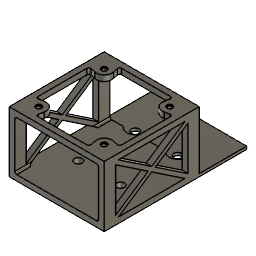
cam_support (Autodesk Fusion 360 design; units mm, degrees)
Autodesk Fusion 360 part; units mm, degrees
sketch "Esboço1" plane through (0, 0, 0) normal (0, 0, 1) x (1, 0, 0)
  line L0 (-20, 37.5) -> (20, 37.5)
  line L1 (25, 32.5) -> (25, -37.5)
  line L2 (25, -37.5) -> (-25, -37.5)
  line L3 (-25, -37.5) -> (-25, 32.5)
  line L4 (-25, 37.5) -> (25, -37.5) construction
  line L5 (25, 37.5) -> (-25, -37.5) construction
  line L6 (-25, 32.5) -> (-25, 37.5)
  line L7 (-20, 37.5) -> (-25, 37.5)
  line L8 (20, 37.5) -> (25, 37.5)
  line L9 (25, 32.5) -> (25, 37.5)
  dimension "d1" = 50
  dimension "d2" = 75
  constraint horizontal L0
  constraint perpendicular L0 L1
  constraint parallel L0 L2
  constraint parallel L1 L3
  constraint coincident L4 origin
  constraint coincident L5 origin
  constraint coincident L4.start L0
  constraint coincident L4.start L3
  constraint coincident L5.start L1
  constraint coincident L5.start L0
  measures "d1" distance of L1.end L2.end
  measures "d2" distance of L5.start L1.end
extrude "Extrusão1" add sketch "Esboço1" along normal blind 32
sketch "Esboço2" plane through (0, 0, 32) normal (0, 0, 1) x (-1, 0, 0)
  line L0 (-25, 37.5) -> (-25, -37.5)
  line L1 (-25, -37.5) -> (25, -37.5)
  line L2 (25, -37.5) -> (25, 37.5)
  line L3 (25, 37.5) -> (-25, 37.5)
  circle A0 centre (11.137, -15) radius 2.05
  circle A1 centre (-11.137, -15) radius 2.05
  circle A2 centre (11.137, 15) radius 2.05
  circle A3 centre (-11.137, 15) radius 2.05
  dimension "d6" = 4.1
  dimension "d7" = 4.1
  dimension "d8" = 4.1
  dimension "d9" = 4.1
  dimension "d10" = 22.274
  dimension "d11" = 13.863
  dimension "d12" = 13.863
  dimension "d13" = 22.274
  dimension "d14" = 30
  dimension "d15" = 22.5
  measures "d6" diameter of A0
  measures "d7" diameter of A1
  measures "d8" diameter of A2
  measures "d9" diameter of A3
  measures "d10" distance of A0.centre A1.centre
  measures "d11" distance of L2 A0.centre
  measures "d12" distance of L2 A2.centre
  measures "d13" distance of A2.centre A3.centre
  measures "d14" distance of A1.centre A3.centre
  measures "d15" distance of L1 A0.centre
extrude "Extrusão2" cut sketch "Esboço2" against normal blind 45 contours A0 | A1 | A2 | A3
ref_plane "Plano de trabalho3" through (0, 47.5, 16) normal (0, 1, 0) x (-1, 0, 0)
sketch "Esboço9" plane through (0, 47.5, 0) normal (0, 1, 0) x (-1, 0, 0)
  line L0 (-25, 0) -> (25, 0)
  line L1 (25, 0) -> (25, 32)
  line L2 (25, 32) -> (-25, 32)
  line L3 (-25, 32) -> (-25, 0)
  line L4 (16.763, 29) -> (-16.763, 29)
  line L5 (-22, 25.7693) -> (-22, 6.2307)
  line L6 (-16.763, 3) -> (16.763, 3)
  line L7 (21, 3) -> (-21, 3)
  line L8 (-22, 4) -> (-22, 28)
  line L9 (-21, 29) -> (21, 29)
  line L10 (22, 28) -> (22, 4)
  arc A0 (-21, 29) -> (-22, 28) centre (-21, 28) ccw
  arc A1 (22, 28) -> (21, 29) centre (21, 28) ccw
  arc A2 (21, 3) -> (22, 4) centre (21, 4) ccw
  arc A3 (-22, 4) -> (-21, 3) centre (-21, 4) ccw
  line L11 (-25, 0) -> (25, 0)
  line L12 (25, 0) -> (25, 32)
  line L13 (25, 32) -> (-25, 32)
  line L14 (-25, 32) -> (-25, 0)
  dimension "d156" = 1
  constraint horizontal L4
  constraint perpendicular L4 L5
  constraint parallel L4 L6
  constraint horizontal L7
  constraint perpendicular L7 L8
  constraint parallel L7 L9
  constraint parallel L8 L10
  constraint tangent L8 A0
  constraint tangent L9 A0
  constraint tangent L9 A1
  constraint tangent L10 A1
  constraint equal A0 A1
  constraint tangent L10 A2
  constraint tangent L7 A2
  constraint equal A0 A2
  constraint tangent L7 A3
  constraint tangent L8 A3
  constraint equal A0 A3
  measures "d156" radius of A0
extrude "Extrusão9" cut sketch "Esboço9" against normal blind 96 contours L4 L5 L6 L7 L8 L9 L10 A0 A1 A2 A3
sketch "Esboço12" plane through (0, 0, 32) normal (0, 0, 1) x (-1, 0, 0)
  circle A0 centre (11.137, -15) radius 2.05
  circle A1 centre (11.137, 15) radius 2.05
  circle A2 centre (-11.137, -15) radius 2.05
  circle A3 centre (-11.137, 15) radius 2.05
  line L0 (-25, 37.5) -> (-25, -37.5)
  line L1 (-25, -37.5) -> (25, -37.5)
  line L2 (25, -37.5) -> (25, 37.5)
  line L3 (25, 37.5) -> (-25, 37.5)
  line L4 (21, 34.5) -> (-21, 34.5)
  line L5 (-22, 33.5) -> (-22, -33.5)
  line L6 (-21, -34.5) -> (21, -34.5)
  line L7 (22, -33.5) -> (22, 33.5)
  line L8 (22, 34.5) -> (-22, -34.5) construction
  line L9 (-22, 34.5) -> (22, -34.5) construction
  arc A4 (-21, 34.5) -> (-22, 33.5) centre (-21, 33.5) ccw
  arc A5 (22, 33.5) -> (21, 34.5) centre (21, 33.5) ccw
  arc A6 (21, -34.5) -> (22, -33.5) centre (21, -33.5) ccw
  arc A7 (-22, -33.5) -> (-21, -34.5) centre (-21, -33.5) ccw
  dimension "d118" = 44
  dimension "d119" = 69
  dimension "d120" = 1
  constraint horizontal L4
  constraint perpendicular L4 L5
  constraint parallel L4 L6
  constraint parallel L5 L7
  constraint coincident L8 origin
  constraint coincident L9 origin
  constraint coincident L9.start L4
  constraint coincident L9.start L5
  constraint tangent L4 A4
  constraint tangent L5 A4
  constraint coincident L8.start L7
  constraint coincident L8.start L4
  constraint tangent L7 A5
  constraint tangent L4 A5
  constraint equal A4 A5
  constraint coincident L9.end L7
  constraint coincident L9.end L6
  constraint tangent L7 A6
  constraint tangent L6 A6
  constraint equal A4 A6
  constraint coincident L8.end L6
  constraint coincident L8.end L5
  constraint tangent L6 A7
  constraint tangent L5 A7
  constraint equal A4 A7
  measures "d118" distance of L8.end L9.end
  measures "d119" distance of L9.start L8.end
  measures "d120" radius of A4
extrude "Extrusão13" cut sketch "Esboço12" against normal blind 5 contours L4 L5 L6 L7 A4 A5 A6 A7
sketch "Esboço13" plane through (0, 0, 32) normal (0, 0, 1) x (-1, 0, 0)
  line L0 (21, -34.5) -> (-21, -34.5)
  arc A0 (-22, -33.5) -> (-21, -34.5) centre (-21, -33.5) ccw
  line L1 (-22, -33.5) -> (-22, 33.5)
  arc A1 (-21, 34.5) -> (-22, 33.5) centre (-21, 33.5) ccw
  line L2 (-21, 34.5) -> (21, 34.5)
  arc A2 (22, 33.5) -> (21, 34.5) centre (21, 33.5) ccw
  line L3 (22, 33.5) -> (22, -33.5)
  arc A3 (21, -34.5) -> (22, -33.5) centre (21, -33.5) ccw
  line L4 (-25, 37.5) -> (-25, -37.5)
  line L5 (-25, -37.5) -> (25, -37.5)
  line L6 (25, -37.5) -> (25, 37.5)
  line L7 (25, 37.5) -> (-25, 37.5)
  circle A4 centre (-17.2, 29.7) radius 1.05
  line L8 (-13.8524, -8.3) -> (-13.2808, -5.5)
  circle A5 centre (-17.2, 29.7) radius 4
  arc A6 (-22, -0.3726) -> (-20.8, -1.3524) centre (-21, -0.3726) ccw
  circle A7 centre (-17.2, -4.7) radius 4
  line L9 (20.8, -1.3524) -> (18, -0.7808)
  line L10 (-22, 25.3726) -> (-22, -0.3726)
  line L11 (12.8726, 34.5) -> (-12.8726, 34.5)
  arc A8 (13.8524, 33.3) -> (12.8726, 34.5) centre (12.8726, 33.5) ccw
  line L12 (20.8, 26.3524) -> (18, 25.7808)
  arc A9 (12.8726, -9.5) -> (13.8524, -8.3) centre (12.8726, -8.5) ccw
  circle A10 centre (17.2, 29.7) radius 4
  line L13 (-20.8, -1.3524) -> (-18, -0.7808)
  arc A11 (25, 32.5) -> (20, 37.5) centre (20, 32.5) ccw
  circle A12 centre (17.2, -4.7) radius 1.05
  line L14 (0, -15) -> (0, 40)
  line L15 (-13.8524, 33.3) -> (-13.2808, 30.5)
  line L16 (-25, 32.5) -> (-25, -17.5)
  line L17 (-12.8726, -9.5) -> (12.8726, -9.5)
  line L18 (-18.25, 30.75) -> (18.25, -5.75) construction
  line L19 (-22, 34.5) -> (22, -9.5) construction
  line L20 (-18.25, -5.75) -> (18.25, -5.75)
  line L21 (22, 34.5) -> (-22, -9.5) construction
  arc A13 (22, 25.3726) -> (20.8, 26.3524) centre (21, 25.3726) ccw
  circle A14 centre (17.2, -4.7) radius 4
  line L22 (22, -0.3726) -> (22, 25.3726)
  line L23 (13.8524, 33.3) -> (13.2808, 30.5)
  circle A15 centre (17.2, 29.7) radius 1.05
  line L24 (18.25, -5.75) -> (18.25, 30.75)
  line L25 (18.25, 30.75) -> (-18.25, 30.75)
  line L26 (18.25, 30.75) -> (-18.25, -5.75) construction
  line L27 (-25, -17.5) -> (25, -17.5)
  arc A16 (-13.8524, -8.3) -> (-12.8726, -9.5) centre (-12.8726, -8.5) ccw
  line L28 (13.8524, -8.3) -> (13.2808, -5.5)
  arc A17 (-20, 37.5) -> (-25, 32.5) centre (-20, 32.5) ccw
  line L29 (25, -17.5) -> (25, 32.5)
  circle A18 centre (-17.2, -4.7) radius 1.05
  line L30 (-20.8, 26.3524) -> (-18, 25.7808)
  line L31 (-18.25, 30.75) -> (-18.25, -5.75)
  arc A19 (20.8, -1.3524) -> (22, -0.3726) centre (21, -0.3726) ccw
  arc A20 (-20.8, 26.3524) -> (-22, 25.3726) centre (-21, 25.3726) ccw
  arc A21 (-12.8726, 34.5) -> (-13.8524, 33.3) centre (-12.8726, 33.5) ccw
  line L32 (44.2599, -12.5) -> (-40.6438, -12.5)
  point P0 (22, -1.5973)
  point P1 (14.0973, -9.5)
  point P2 (-22, 26.5973)
  point P3 (22, 26.5973)
  point P4 (14.0973, 34.5)
  point P5 (-22, -1.5973)
  point P6 (-14.0973, -9.5)
  point P7 (0, 12.5)
  point P8 (0, -15)
  point P9 (0, 12.5)
  point P10 (-14.0973, 34.5)
  dimension "d123" = 36.5
  dimension "d124" = 36.5
  dimension "d125" = 2.1
  dimension "d126" = 2.1
  dimension "d127" = 2.1
  dimension "d128" = 2.1
  dimension "d129" = 44
  dimension "d130" = 44
  dimension "d131" = 8
  dimension "d132" = 8
  dimension "d133" = 8
  dimension "d134" = 8
  dimension "d135" = 4
  dimension "d136" = 4
  dimension "d137" = 4
  dimension "d138" = 4
  dimension "d139" = 4
  dimension "d140" = 4
  dimension "d141" = 4
  dimension "d142" = 4
  dimension "d143" = 1
  dimension "d144" = 3
  dimension "d145" = 3
  constraint horizontal L25
  constraint perpendicular L25 L31
  constraint parallel L20 L25
  constraint parallel L24 L31
  constraint coincident P9 L26
  constraint coincident P9 L18
  constraint coincident A4.centre L18
  constraint coincident A10.centre L26
  constraint coincident A12.centre L18
  constraint coincident A7.centre L26
  constraint coincident P8 L14.start
  constraint midpoint L14 L26
  constraint tangent A4 L25
  constraint tangent A15 L25
  constraint tangent A12 L24
  constraint tangent A18 L31
  constraint horizontal L11
  constraint perpendicular L10 L11
  constraint parallel L11 L17
  constraint parallel L10 L22
  constraint coincident P9 L21
  constraint coincident P9 L19
  constraint coincident P9 P7
  constraint concentric A10 A15
  constraint concentric A12 A14
  constraint concentric A7 A18
  constraint concentric A4 A5
  constraint coincident P10 L11
  constraint coincident L15.end A5
  constraint tangent A5 L15
  constraint coincident P2 L10
  constraint coincident L30.end A5
  constraint tangent A5 L30
  constraint coincident P4 L11
  constraint coincident L23.end A10
  constraint tangent A10 L23
  constraint coincident P3 L22
  constraint coincident L12.end A10
  constraint tangent L12 A10
  constraint coincident P0 L22
  constraint coincident L9.end A14
  constraint tangent L9 A14
  constraint coincident P1 L17
  constraint coincident L28.end A14
  constraint tangent A14 L28
  constraint coincident P6 L17
  constraint coincident L8.end A7
  constraint tangent L8 A7
  constraint coincident P5 L10
  constraint coincident L13.end A7
  constraint tangent A7 L13
  constraint coincident P10 L15
  constraint coincident L19.start L11
  constraint tangent L15 A21
  constraint tangent L11 A21
  constraint coincident P4 L23
  constraint coincident L21.start L11
  constraint tangent A8 L23
  constraint tangent L11 A8
  constraint equal A8 A21
  constraint coincident L19.start L10
  constraint coincident P2 L30
  constraint tangent L10 A20
  constraint tangent L30 A20
  constraint equal A20 A21
  constraint coincident P5 L13
  constraint coincident L21.end L10
  constraint tangent A6 L13
  constraint tangent A6 L10
  constraint equal A6 A21
  constraint coincident L21.end L17
  constraint coincident P6 L8
  constraint tangent L17 A16
  constraint tangent L8 A16
  constraint equal A16 A21
  constraint coincident P1 L28
  constraint coincident L19.end L17
  constraint tangent A9 L28
  constraint tangent A9 L17
  constraint equal A9 A21
  constraint coincident P0 L9
  constraint coincident L19.end L22
  constraint tangent L9 A19
  constraint tangent L22 A19
  constraint equal A19 A21
  constraint coincident L21.start L22
  constraint coincident P3 L12
  constraint tangent A13 L22
  constraint tangent L12 A13
  constraint equal A13 A21
  constraint perpendicular L4 L32
  measures "d123" distance of L18.end L20.start
  measures "d124" distance of L20.start L18.start
  measures "d125" diameter of A4
  measures "d126" diameter of A15
  measures "d127" diameter of A12
  measures "d128" diameter of A18
  measures "d129" distance of L19.end L21.end
  measures "d130" distance of L19.start L21.end
  measures "d131" diameter of A10
  measures "d132" diameter of A14
  measures "d133" diameter of A7
  measures "d134" diameter of A5
  measures "d135" horizontal distance of L13.end P5
  measures "d136" vertical distance of L8.end P6
  measures "d137" vertical distance of P1 L28.end
  measures "d138" horizontal distance of P0 L9.end
  measures "d139" horizontal distance of L12.end P3
  measures "d140" vertical distance of L23.end P4
  measures "d141" vertical distance of P10 L15.end
  measures "d142" horizontal distance of P2 L30.end
  measures "d143" radius of A21
  measures "d144" distance of L7 L11
  measures "d145" distance of L17 L32
extrude "Extrusão14" add sketch "Esboço13" against normal blind 3 contours L3 L9 A9 L14 L17 L20 A14 L24 L28 A19 L32 | L2 A2 L3 L6 L7 L11 A11 L14 L22 L29 L32 | L1 A1 L2 L4 L7 L10 L11 L14 L16 A17 L32 | L1 L8 A6 A7 L13 L14 L17 L20 A16 L31 L32 | L2 A2 L3 A8 L12 A10 A13 L23 L24 L25 | L1 A1 L2 A5 L15 L25 L30 L31 A20 A21 | A12 L20 A14 L24 | L20 A14 L24 | A7 L20 A18 L31 | A7 L20 L31 | A10 A15 L24 L25 | A10 L24 L25 | A12 L20 L24 | A4 A5 L25 L31 | A5 L25 L31 | L20 A18 L31 | A15 L24 L25 | A4 L25 L31
sketch "Esboço14" plane through (0, 0, 32) normal (0, 0, 1) x (-1, 0, 0)
  line L0 (22, -12.5) -> (22, -33.5)
  arc A0 (21, -34.5) -> (22, -33.5) centre (21, -33.5) ccw
  line L1 (21, -34.5) -> (-21, -34.5)
  arc A1 (-22, -33.5) -> (-21, -34.5) centre (-21, -33.5) ccw
  line L2 (-22, -33.5) -> (-22, -12.5)
  line L3 (-22, -12.5) -> (22, -12.5)
  circle A2 centre (17.2, -4.7) radius 1.05
  circle A3 centre (-17.2, -4.7) radius 1.05
  circle A4 centre (17.2, 29.7) radius 1.05
  circle A5 centre (-17.2, 29.7) radius 1.05
  arc A6 (20.8, -1.3524) -> (22, -0.3726) centre (21, -0.3726) ccw
  line L4 (20.8, -1.3524) -> (18.25, -0.8318)
  line L5 (18.25, -0.8318) -> (18.25, -0.8403)
  arc A7 (18.25, -0.8403) -> (13.3403, -5.75) centre (17.2, -4.7) ccw
  line L6 (13.3403, -5.75) -> (13.3318, -5.75)
  line L7 (13.3318, -5.75) -> (13.8524, -8.3)
  arc A8 (12.8726, -9.5) -> (13.8524, -8.3) centre (12.8726, -8.5) ccw
  line L8 (12.8726, -9.5) -> (-12.8726, -9.5)
  arc A9 (-13.8524, -8.3) -> (-12.8726, -9.5) centre (-12.8726, -8.5) ccw
  line L9 (-13.8524, -8.3) -> (-13.3318, -5.75)
  line L10 (-13.3318, -5.75) -> (-13.3403, -5.75)
  arc A10 (-13.3403, -5.75) -> (-18.25, -0.8403) centre (-17.2, -4.7) ccw
  line L11 (-18.25, -0.8403) -> (-18.25, -0.8318)
  line L12 (-18.25, -0.8318) -> (-20.8, -1.3524)
  arc A11 (-22, -0.3726) -> (-20.8, -1.3524) centre (-21, -0.3726) ccw
  line L13 (-22, -0.3726) -> (-22, 25.3726)
  arc A12 (-20.8, 26.3524) -> (-22, 25.3726) centre (-21, 25.3726) ccw
  line L14 (-20.8, 26.3524) -> (-18.25, 25.8318)
  line L15 (-18.25, 25.8318) -> (-18.25, 25.8403)
  arc A13 (-18.25, 25.8403) -> (-13.3403, 30.75) centre (-17.2, 29.7) ccw
  line L16 (-13.3403, 30.75) -> (-13.3318, 30.75)
  line L17 (-13.3318, 30.75) -> (-13.8524, 33.3)
  arc A14 (-12.8726, 34.5) -> (-13.8524, 33.3) centre (-12.8726, 33.5) ccw
  line L18 (-12.8726, 34.5) -> (12.8726, 34.5)
  arc A15 (13.8524, 33.3) -> (12.8726, 34.5) centre (12.8726, 33.5) ccw
  line L19 (13.8524, 33.3) -> (13.3318, 30.75)
  line L20 (13.3318, 30.75) -> (13.3403, 30.75)
  arc A16 (13.3403, 30.75) -> (18.25, 25.8403) centre (17.2, 29.7) ccw
  line L21 (18.25, 25.8403) -> (18.25, 25.8318)
  line L22 (18.25, 25.8318) -> (20.8, 26.3524)
  arc A17 (22, 25.3726) -> (20.8, 26.3524) centre (21, 25.3726) ccw
  line L23 (22, 25.3726) -> (22, -0.3726)
  line L24 (25, -37.5) -> (25, 37.5)
  line L25 (25, 37.5) -> (-25, 37.5)
  line L26 (-25, 37.5) -> (-25, -37.5)
  line L27 (-25, -37.5) -> (25, -37.5)
  circle A18 centre (17.2, 29.7) radius 1.5
  circle A19 centre (17.2, -4.7) radius 1.5
  circle A20 centre (-17.2, -4.7) radius 1.5
  circle A21 centre (-17.2, 29.7) radius 1.5
  dimension "d150" = 3
  dimension "d151" = 3
  dimension "d152" = 3
  dimension "d153" = 3
  constraint concentric A4 A18
  constraint concentric A2 A19
  constraint concentric A3 A20
  constraint concentric A5 A21
  measures "d150" diameter of A18
  measures "d151" diameter of A19
  measures "d152" diameter of A20
  measures "d153" diameter of A21
extrude "Extrusão15" cut sketch "Esboço14" against normal blind 0.5 contours A18 | A19 | A20 | A21
sketch "Esboço15" plane through (-25, 0, 0) normal (-1, 0, 0) x (0, -1, 0)
  line L0 (37.5, 32) -> (-37.5, 32)
  line L1 (-37.5, 32) -> (-37.5, 0)
  line L2 (-37.5, 0) -> (37.5, 0)
  line L3 (37.5, 0) -> (37.5, 32)
  line L4 (-9.5, 32) -> (34.5, 32)
  line L5 (34.5, 32) -> (34.5, 0)
  line L6 (34.5, 0) -> (-9.5, 0)
  line L7 (-9.5, 0) -> (-9.5, 32)
  line L8 (31.5, 29) -> (-6.5, 29)
  line L9 (-6.5, 29) -> (-6.5, 3)
  line L10 (-6.5, 3) -> (31.5, 3)
  line L11 (31.5, 3) -> (31.5, 29)
  line L12 (31.5, 29) -> (-6.5, 3) construction
  line L13 (-6.5, 29) -> (31.5, 3) construction
  circle A0 centre (-6.5, 29) radius 1.5
  circle A1 centre (31.5, 29) radius 1.5
  circle A2 centre (31.5, 3) radius 1.5
  circle A3 centre (-6.5, 3) radius 1.5
  line L14 (-5, 3) -> (31.5, 27.5)
  line L15 (-6.5, 4.5) -> (30, 29)
  line L16 (-5, 29) -> (31.5, 4.5)
  line L17 (30, 3) -> (-6.5, 27.5)
  line L18 (-12.5, 32) -> (-42.5, 32)
  line L19 (-42.5, 32) -> (-42.5, 1.5)
  line L20 (-42.5, 1.5) -> (-12.5, 1.5)
  line L21 (-12.5, 1.5) -> (-12.5, 32)
  point P0 (-9.5, 32)
  point P1 (34.5, 32)
  point P2 (12.5, 16)
  point P3 (-12.5, 32)
  dimension "d158" = 44
  dimension "d159" = 32
  dimension "d160" = 38
  dimension "d162" = 3
  dimension "d163" = 3
  dimension "d164" = 3
  dimension "d165" = 3
  dimension "d172" = 30
  dimension "d173" = 30.5
  constraint horizontal L4
  constraint vertical L5
  constraint horizontal L6
  constraint vertical L7
  constraint coincident L2 L5.end
  constraint coincident P0 L4.start
  constraint horizontal L8
  constraint perpendicular L8 L9
  constraint parallel L8 L10
  constraint parallel L9 L11
  constraint coincident L12 P2
  constraint coincident L13 P2
  constraint coincident L8.end L9.start
  constraint coincident L8.start L11.end
  constraint coincident L10.end L11.start
  constraint coincident L9.end L10.start
  constraint coincident A3 L14.start
  constraint coincident L10 L14.start
  constraint coincident A1 L14.end
  constraint coincident L11 L14.end
  constraint coincident A3 L15.start
  constraint coincident L9 L15.start
  constraint coincident A1 L15.end
  constraint coincident L8 L15.end
  constraint coincident A0 L16.start
  constraint coincident L8 L16.start
  constraint coincident A2 L16.end
  constraint coincident L11 L16.end
  constraint coincident A2 L17.start
  constraint coincident L10 L17.start
  constraint coincident L9 L17.end
  constraint coincident A0 L17.end
  constraint horizontal L18
  constraint vertical L19
  constraint horizontal L20
  constraint vertical L21
  constraint coincident P3 L18.start
  measures "d158" distance of P0 P1
  measures "d159" distance of P0 L6.end
  measures "d160" distance of L9.end L10.end
  measures "d162" diameter of A0
  measures "d163" diameter of A1
  measures "d164" diameter of A2
  measures "d165" diameter of A3
  measures "d172" distance of P3 L18.end
  measures "d173" distance of P3 L20.end
extrude "Extrusão16" cut sketch "Esboço15" against normal blind 60 contours L0 L1 L18 L20 L21 | L8 L15 L16 | L11 L14 L16 | L9 L15 L17 | L10 L14 L17
sketch "Esboço16" plane through (0, 0, 1.5) normal (0, 0, 1) x (-1, 0, 0)
  line L0 (-25, -12.5) -> (-25, -37.5)
  line L1 (-25, -37.5) -> (25, -37.5)
  line L2 (25, -37.5) -> (25, -12.5)
  line L3 (25, -12.5) -> (-25, -12.5)
  circle A0 centre (-11.137, -15) radius 2.05
  circle A1 centre (11.137, -15) radius 2.05
  circle A2 centre (-11.137, -15) radius 4.5
  circle A3 centre (11.137, -15) radius 4.5
  dimension "d174" = 9
  dimension "d175" = 9
  constraint concentric A0 A2
  constraint concentric A1 A3
  measures "d174" diameter of A2
  measures "d175" diameter of A3
extrude "Extrusão17" cut sketch "Esboço16" along normal blind 3 contours L3 A2 | L3 A3 picked at (-11.703, -11.4131) picked at (10.2449, -11.6515)
